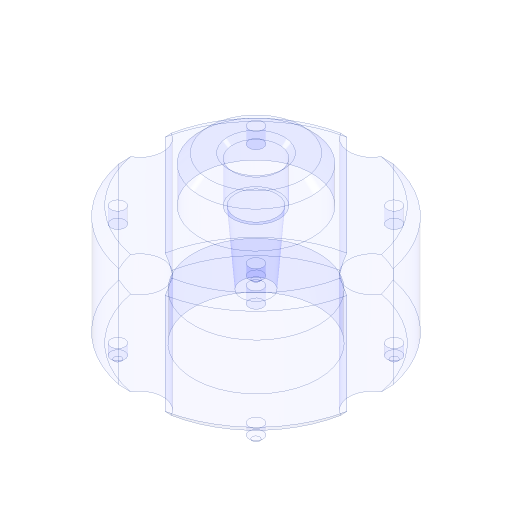
# Autodesk Inventor part: cpd_lowrcf_1.3_p2_20230620
Saved by Autodesk Inventor 2024 (Build 280153000, 153)
## iProperties
Created: 2021-12-08
Part Number: cpd_lowrcf_1.3_p2_20230620
Material: Generic
Document SubType Name: Modeling
Designer: tomos
Density: 1 g/cm^3
Appearance: Clear - Blue
Author: tomos
Autodesk Inventor part; units mm, degrees
ref_plane "YZ Plane" through (0, 0, 0) normal (1, 0, 0) x (0, 1, 0)
ref_plane "XZ Plane" through (0, 0, 0) normal (0, 1, 0) x (-1, 0, 0)
ref_plane "XY Plane" through (0, 0, 0) normal (0, 0, 1) x (1, 0, 0)
sketch "Sketch1" plane through (0, 0, 0) normal (0, 0, 1) x (1, 0, 0)
  line L0 (0, 0) -> (0, 19.4488) construction
  line L1 (0, 0) -> (15.8946, 0) construction
  line L2 (1.61, 5) -> (6.7, 5)
  line L3 (6.7, 5) -> (6.7, 0)
  line L4 (6.7, 0) -> (12.5, 0)
  line L5 (12.5, 0) -> (12.5, 12.791)
  line L6 (1.0049, 10.15) -> (0.7849, 10.15) construction
  line L7 (1.6103, 4.761) -> (2.6467, 18.8742) construction
  line L8 (0.4645, 3.15) -> (0.2, 3.15) construction
  line L9 (0, 2.7) -> (1.1563, 2.7) construction
  line L10 (12.5, 12.791) -> (2.2, 12.791)
  line L11 (2.2, 12.791) -> (1.61, 5)
  point P0 (9.6, 0)
  dimension "d1" = 12.5
  dimension "d2" = 6.7
  dimension "d7" = 5
  dimension "d53" = 0.22
  dimension "d55" = 0.2
  dimension "d58" = 2.3
  dimension "d62" = 1.61
  dimension "d63" = 2.2
  dimension "d64" = 12.791
  constraints: 24 end point, 5 horizontal, 4 point on line, 2 perpendicular, 2 vertical, 1 midpoint
  measures "d1" distance between parallel lines of L5 L0
  measures "d2" distance between parallel lines of L3 L0
  measures "d7" distance between parallel lines of L2 L1
  measures "d53" distance of L6.start L6.end
  measures "d55" distance from line of L0 L8.end
  measures "d58" distance between parallel lines of L2 L9
  measures "d62" distance from line of L0 L2.start
  measures "d63" distance from line of L0 L10.end
  measures "d64" distance from line of point (9.6, 0) L10
revolve "Revolution1" add sketch "Sketch1" angle 360 about axis through (0, 0, 0) along (0, 1, 0)
chamfer "Chamfer2" distance 1 angle 45 2 edges at (-12.5, 0, 0) (-12.5, 12.791, 0)
sketch "Sketch7" plane through (0, 12.791, 0) normal (0, 1, 0) x (1, 0, 0)
  circle A0 centre (0, 0) radius 10.5 construction
  line L0 (0, 0) -> (23.4924, 0) construction
  line L1 (0, 0) -> (0, 17.9898) construction
  line L2 (0, 0) -> (-15.6301, 15.6301) construction
  circle A1 centre (-7.4246, 7.4246) radius 0.75
  point P0 (12.4999, 0)
  dimension "d84" = 21
  dimension "d85" = 45
  dimension "d86" = 1.5
  constraints: 6 end point, 2 point on line, 1 centre point, 1 coincident, 1 horizontal, 1 vertical, 3 other
  measures "d85" angle of L1 L2
  measures "d86" diameter of A1
extrude "Extrusion6" cut sketch "Sketch7" against normal blind 1.7
sketch "Sketch8" plane through (0, 12.791, 0) normal (0, 1, 0) x (1, 0, 0)
  circle A0 centre (0, 0) radius 12.5 construction
  line L0 (0, 0) -> (0, 17.9558) construction
  circle A1 centre (0, 12.5) radius 2.5
  dimension "d89" = 25
  dimension "d90" = 5
  constraints: 2 end point, 1 centre point, 1 coincident, 1 point on line, 1 vertical, 1 vertical alignment, 2 other
  measures "d90" diameter of A1
extrude "Extrusion7" cut sketch "Sketch8" against normal blind 12.791
pattern_circular "Circular Pattern4" count 4 over 360 about axis through (0, 8.8955, 0) along (0, -1, 0) of "Extrusion6", "Extrusion7"
sketch "Sketch9" plane through (0, 12.791, -12.5) normal (0, 1, 0) x (1, 0, 0)
  circle A0 centre (0, -12.5) radius 6
  circle A1 centre (0, -12.5) radius 2.5
  dimension "d96" = 12
  dimension "d97" = 5
  constraints: 2 centre point, 2 coincident
  measures "d96" diameter of A0
  measures "d97" diameter of A1
extrude "Extrusion8" add sketch "Sketch9" along normal blind 4.9
chamfer "Chamfer7" distance 1 angle 45 1 edges at (-6, 17.691, 0)
chamfer "Chamfer8" distance 0.5 angle 45 1 edges at (-2.5, 17.691, 0)
sketch "Sketch10" plane through (0, 0, -12.5) normal (0, -1, 0) x (1, 0, 0)
  circle A0 centre (0, 12.5) radius 10.5 construction
  line L0 (0, 12.5) -> (14.2322, 12.5) construction
  line L1 (0, 12.5) -> (13.4469, 25.9469) construction
  circle A1 centre (7.4246, 19.9246) radius 0.75
  dimension "d106" = 21
  dimension "d107" = 45
  dimension "d108" = 1.5
  constraints: 4 end point, 1 centre point, 1 coincident, 1 horizontal, 1 point on line, 3 other
  measures "d107" angle of L0 L1
  measures "d108" diameter of A1
extrude "Extrusion9" add sketch "Sketch10" along normal blind 1.5
chamfer "Chamfer9" distance 0.35 angle 45 1 edges at (6.6746, -1.5, 7.4246)
pattern_circular "Circular Pattern5" count 4 over 360 about axis through (0, 2.5, 0) along (0, -1, 0) of "Extrusion9", "Chamfer9"
equation "\"cutpipette_length\" = 5.7"
body "Solid1"
